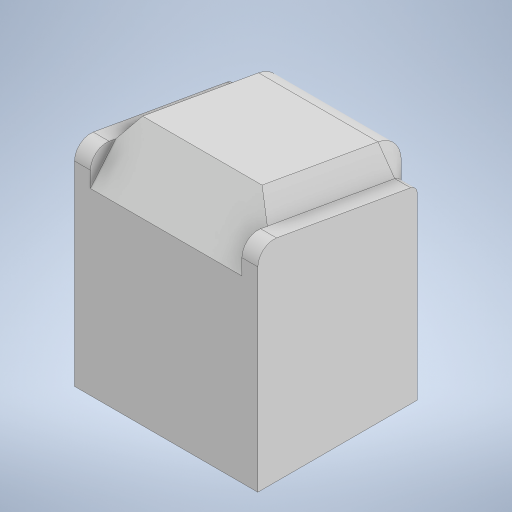
# Autodesk Inventor part: RevII Printer Envelope Study
Saved by Autodesk Inventor 2024 (Build 280153000, 153)
## iProperties
Created: 2024-07-22
Part Number: RevII Printer Envelope Study
Material: Generic
Document SubType Name: Modeling
Designer: Ishaan
Density: 1 g/cm^3
Appearance: Default
Author: Ishaan
Autodesk Inventor part; units mm, degrees
ref_plane "YZ Plane" through (0, 0, 0) normal (1, 0, 0) x (0, 1, 0)
sketch "Sketch1" plane through (0, 0, 0) normal (0, 0, 1) x (1, 0, 0)
  line L0 (230, -200) -> (-230, -200)
  line L1 (-230, -200) -> (-230, 200)
  line L2 (-230, 200) -> (230, 200)
  line L3 (230, 200) -> (230, -200)
  line L4 (230, -200) -> (-230, 200) construction
  line L5 (-230, -200) -> (230, 200) construction
  line L6 (-190, 200) -> (-160.6372, 250.8579)
  line L7 (-160.6372, 250.8579) -> (139.1421, 250.8579)
  line L8 (139.1421, 250.8579) -> (190, 200)
  line L9 (139.1421, 250.8579) -> (122.8634, 211.5574) construction
  line L10 (135, 250.8579) -> (135, 240.8579) construction
  line L11 (230, 200) -> (190, 200)
  line L12 (190, 200) -> (190, 160)
  line L13 (190, 160) -> (230, 160)
  line L14 (230, 160) -> (230, 200)
  line L15 (-150, 110) -> (150, 110)
  line L16 (150, 110) -> (150, -140)
  line L17 (150, -140) -> (-150, -140)
  line L18 (-150, -140) -> (-150, 110)
  line L19 (-230, -200) -> (-190, -200)
  line L20 (-190, -200) -> (-190, -160)
  line L21 (-190, -160) -> (-230, -160)
  line L22 (-230, -160) -> (-230, -200)
  line L23 (230, -200) -> (190, -200)
  line L24 (190, -200) -> (190, -160)
  line L25 (190, -160) -> (230, -160)
  line L26 (230, -160) -> (230, -200)
  line L27 (-230, 200) -> (-190, 200)
  line L28 (-190, 200) -> (-190, 160)
  line L29 (-190, 160) -> (-230, 160)
  line L30 (-230, 160) -> (-230, 200)
  line L31 (-40, 200) -> (40, 200)
  line L32 (40, 200) -> (40, 160)
  line L33 (40, 160) -> (-40, 160)
  line L34 (-40, 160) -> (-40, 200)
  line L35 (125, 250.8579) -> (135, 250.8579)
  line L36 (135, 250.8579) -> (135, 230.8579)
  line L37 (135, 230.8579) -> (125, 230.8579)
  line L38 (125, 230.8579) -> (125, 250.8579)
  line L39 (149.1421, 240.8579) -> (142.0711, 247.9289)
  line L40 (142.0711, 247.9289) -> (127.9289, 233.7868)
  line L41 (127.9289, 233.7868) -> (134.2929, 227.4228)
  line L42 (135.7071, 227.4228) -> (149.1421, 240.8579)
  line L43 (135, 200) -> (132, 200)
  line L44 (132, 200) -> (132, 239)
  line L45 (132, 239) -> (135, 239)
  line L46 (135, 239) -> (135, 200)
  line L47 (135, 200) -> (95, 200)
  line L48 (95, 200) -> (95, 180)
  line L49 (95, 180) -> (135, 180)
  line L50 (135, 180) -> (135, 200)
  line L51 (-222, 80) -> (-132, 80)
  line L52 (-132, 80) -> (-132, -140)
  line L53 (-132, -140) -> (-222, -140)
  line L54 (-222, -140) -> (-222, 80)
  circle A0 centre (-112, -40) radius 100
  circle A1 centre (112, -40) radius 100
  line L55 (-230, -40) -> (230, -40) construction
  line L56 (-112, -40) -> (112, -40)
  arc A2 (134.2929, 227.4228) -> (135.7071, 227.4228) centre (135, 228.1299) ccw
  point P0 (0, 0)
  point P1 (0, 110)
  point P2 (0, 200)
  point P3 (135, 226.7157)
  point P4 (0, -40)
  dimension "d0" = 460
  dimension "d1" = 400
  dimension "d2" = 40
  dimension "d3" = 40
  dimension "d4" = 120
  dimension "d5" = 135
  dimension "d30" = 67.5
  dimension "d32" = 10
  dimension "d34" = 50.8579
  dimension "d35" = 40
  dimension "d36" = 40
  dimension "d37" = 300
  dimension "d38" = 250
  dimension "d39" = 60
  dimension "d40" = 40
  dimension "d41" = 40
  dimension "d42" = 40
  dimension "d43" = 40
  dimension "d44" = 40
  dimension "d45" = 40
  dimension "d46" = 80
  dimension "d47" = 40
  dimension "d48" = 10
  dimension "d50" = 10
  dimension "d51" = 3
  dimension "d52" = 39
  dimension "d53" = 40
  dimension "d54" = 20
  dimension "d55" = 55
  dimension "d56" = 105
  dimension "d57" = 90
  dimension "d58" = 220
  dimension "d59" = 8
  dimension "d60" = 20
  dimension "d61" = 55
  dimension "d63" = 200
  dimension "d64" = 160
  dimension "d65" = 118
  dimension "d66" = 1
  constraints: 114 end point, 24 parallel, 15 perpendicular, 14 point on line, 12 horizontal, 9 midpoint, 3 centre point, 2 point on circle, 2 tangent, 1 equal radius, 1 vertical, 1 vertical alignment
  measures "d0" distance of L1.end L2.end
  measures "d1" distance of L0.end L1.end
  measures "d2" distance from line of L3 L8.end
  measures "d3" distance from line of L6.start L1
  measures "d4" angle of L7 L6
  measures "d5" angle of L8 L7
  measures "d30" angle of L9 L7
  measures "d32" distance of L10.end L10.start
  measures "d34" distance between parallel lines of L2 L7
  measures "d35" distance of L13.end L12.end
  measures "d36" distance of L12.end L11.end
  measures "d37" distance of L16.end L17.end
  measures "d38" distance of L15.end L16.end
  measures "d39" distance between parallel lines of L0 L17
  measures "d40" distance of L21.end L20.end
  measures "d41" distance of L20.end L19.end
  measures "d42" distance of L24.end L25.end
  measures "d43" distance of L23.end L24.end
  measures "d44" distance of L28.end L29.end
  measures "d45" distance of L27.end L28.end
  measures "d46" distance of L32.end L33.end
  measures "d47" distance of L31.end L32.end
  measures "d48" distance of L36.end L37.end
  measures "d50" distance of L40.end point (135, 226.716)
  measures "d51" distance of L44.end L45.end
  measures "d52" distance of L45.end L43.start
  measures "d53" distance of L49.end L48.end
  measures "d54" distance of L48.end L47.end
  measures "d55" distance between parallel lines of L48 L32
  measures "d56" distance between parallel lines of L3 L38
  measures "d57" distance of L52.end L53.end
  measures "d58" distance of L51.end L52.end
  measures "d59" distance between parallel lines of L1 L54
  measures "d60" distance between parallel lines of L21 L53
  measures "d61" distance between parallel lines of L12 L50
  measures "d63" diameter of A1
  measures "d64" distance between parallel lines of L0 L56
  measures "d65" distance from line of L56.start L1
  measures "d66" radius of A2
extrude "Extrusion1" add sketch "Sketch1" along normal blind 450 contours L0 L24 L25 L3 | L0 L20 L21 L1 L29 L28 L2 L34 L33 L32 L48 L49 L50 L12 L13 L3 L25 L24 | L0 L1 L21 L20 | L13 L12 L2 L3 | L2 L46 A2 L42 L8 | L1 L2 L28 L29 | L50 L49 L48 L2 | L2 L44 L41 A2 L46 | L42 A2 L46 L36 L40 L8 | L2 L6 L7 L38 L37 L41 L44 | A2 L41 L44 L37 L46 | L40 L36 L7 L8 | L41 L37 L44 | L37 L44 L40 L45 L36 | L40 L45 L44 L41 L37 L38 L7 L36 | L36 L45 L40 | L2 L32 L33 L34 | L41 L40 L44 L37 | L40 L44 L45 | L15 L16 A1 L56 A0 L52 L51 L18 | L51 L52 A0 L18 | L18 A0 L53 L54 L51 | A1 L16 | L16 A1 | A0 L52 L18 | L18 A0 | L16 L17 A1 | A1 L17 A0 L56 | A0 L52 L17 L18 | A0 L52 | A0 L17 L52
sketch "Sketch2" plane through (0, 0, 450) normal (0, 0, 1) x (1, 0, 0)
  line L0 (-160.6372, 250.8579) -> (-190, 200) projected
  line L1 (-190, 200) -> (-230, 200) projected
  line L2 (-230, 200) -> (-230, -200) projected
  line L3 (-230, -200) -> (230, -200) projected
  line L4 (230, -200) -> (230, 200) projected
  line L5 (230, 200) -> (190, 200) projected
  line L6 (190, 200) -> (139.1421, 250.8579) projected
  line L7 (139.1421, 250.8579) -> (-160.6372, 250.8579) projected
  line L8 (230, 180) -> (-230, 180)
  point P0 (0, 0)
  dimension "d9" = 20
  constraints: 2 end point, 2 point on line
  measures "d9" distance between parallel lines of L8 L1
revolve "Revolution1" add sketch "Sketch2" angle 80 about axis through (230, 180, 450) along (1, 0, 0) contours L7 L6 L5 L4 L8 L2 L1 L0
sketch "Sketch3" plane through (-230, 180, 450) normal (0, -0.9848078, 0.1736482) x (1, 0, 0)
  line L0 (0, 20) -> (0, 0) projected
  line L1 (460, 0) -> (0, 0) projected
  line L2 (460, 0) -> (460, 20) projected
  line L3 (460, 20) -> (420, 20) projected
  line L4 (420, 20) -> (369.1421, 70.8579) projected
  line L5 (369.1421, 70.8579) -> (69.3628, 70.8579) projected
  line L6 (69.3628, 70.8579) -> (40, 20) projected
  line L7 (40, 20) -> (0, 20) projected
  point P0 (230, -474.4202)
ref_plane "Work Plane4" through (-230, -208.6603, 455) normal (0, 0.8660254, -0.5) x (1, 0, 0)
ref_plane "Work Plane3" through (-230, -200, 450) normal (0, 0.8660254, -0.5) x (1, 0, 0)
sketch "Sketch7" plane through (230, -200, 0) normal (1, 0, 0) x (0, 0, -1)
  line L0 (0, 0) -> (0, 400) projected
  line L1 (0, 400) -> (-450, 400) projected
  arc A0 (-450, 400) -> (-469.6962, 383.473) centre (-450, 380) ccw projected
  line L2 (-450, 380) -> (-469.6962, 383.473) projected
  line L3 (-450, 0) -> (-450, 380) projected
  line L4 (0, 0) -> (-450, 0) projected
  line L5 (-450, 0) -> (-537.3128, 0)
  line L6 (-537.3128, 0) -> (-469.6962, 383.473)
  arc A1 (-450, 400) -> (-469.6962, 383.473) centre (-450, 380) ccw projected
  line L7 (-450, 380) -> (-469.6962, 383.473) projected
  point P0 (0, 200)
  constraints: 4 end point, 1 horizontal, 1 perpendicular, 1 point on circle, 1 tangent
extrude "Extrusion7" add sketch "Sketch7" against normal blind 40 contours L5 L6 L2 L3
fillet "Fillet6" radius 40 1 edges at (210, -200, 537.3128)
mirror "Mirror1" about plane through (0, 0, 0) normal (1, 0, 0) of "Extrusion7", "Fillet6"
ref_plane "Work Plane5" through (-230, -200, 450) normal (0, 0.7660444, -0.6427876) x (1, 0, 0)
sketch "Sketch9" plane through (-160.6372, 192.3043, 519.7814) normal (0, -0.9848078, 0.1736482) x (1, 0, 0)
  line L0 (-29.3628, -50.8579) -> (-29.3628, -70.8579) projected
  line L1 (350.6372, -70.8579) -> (-29.3628, -70.8579) projected
  line L2 (350.6372, -70.8579) -> (350.6372, -50.8579) projected
  line L3 (350.6372, -50.8579) -> (299.7793, 0) projected
  line L4 (299.7793, 0) -> (0, 0) projected
  line L5 (0, 0) -> (-29.3628, -50.8579) projected
  point P0 (160.6372, -545.278)
extrude "Extrusion8" add sketch "Sketch9" along normal up to surface surface through (-230, -200, 450) normal (0, 0.7660444, -0.6427876)
sketch "Sketch11" plane through (190, -200, 0) normal (-1, 0, 0) x (0, 0, 1)
  line L0 (526.0594, 63.8214) -> (508.3683, 48.9768) projected
  line L1 (508.3683, 48.9768) -> (450, 380) projected
  line L2 (450, 0) -> (450, 380) projected
  line L3 (450, 0) -> (489.6426, 0) projected
  arc A0 (489.6426, 0) -> (529.035, 46.9459) centre (489.6426, 40) ccw projected
  line L4 (529.035, 46.9459) -> (526.0594, 63.8214) projected
  line L5 (508.4341, 49.0321) -> (450, 0)
  point P0 (0, 200)
  point P1 (508.3683, 48.9768)
  constraints: 2 end point, 1 collinear
extrude "Extrusion9" add sketch "Sketch11" along normal up to next contours L5 L2 L1
sketch "Sketch6" plane through (-230, -200, 0) normal (-1, 0, 0) x (0, 0, 1)
  line L0 (0, 400) -> (0, 0) projected
  line L1 (0, 0) -> (450, 0) projected
  line L2 (450, 380) -> (450, 0) projected
  line L3 (450, 380) -> (512.6612, 24.6305) projected
  line L4 (531.0933, 35.2723) -> (512.6612, 24.6305) projected
  line L5 (469.6962, 383.473) -> (531.0933, 35.2723) projected
  arc A0 (469.6962, 383.473) -> (450, 400) centre (450, 380) ccw projected
  line L6 (0, 400) -> (450, 400) projected
  line L7 (512.6612, 24.6305) -> (470, 0)
  line L8 (470, 0) -> (450, 0)
  point P0 (0, 200)
  constraints: 4 end point, 1 collinear, 1 horizontal
equation "\"d30\" = 0.5 * d5"
body "Solid1"
